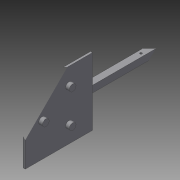
# Autodesk Inventor part: Arm_Base-Rod-Rev2
Saved by Autodesk Inventor 2015 (Build 190159000, 159)
## iProperties
Created: 2016-12-23
Part Number: Arm_Base-Rod-Rev2
Material: Generic
Document SubType Name: Modeling
Designer: Guy
Density: 1 g/cm^3
Appearance: Default
Author: Guy
Autodesk Inventor part; units mm, degrees
ref_plane "YZ Plane" through (0, 0, 0) normal (1, 0, 0) x (0, 1, 0)
ref_plane "XZ Plane" through (0, 0, 0) normal (0, 1, 0) x (-1, 0, 0)
ref_plane "XY Plane" through (0, 0, 0) normal (0, 0, 1) x (1, 0, 0)
sketch "Sketch1" plane through (0, 0, 0) normal (1, 0, 0) x (0, 1, 0)
  line L0 (0, 0) -> (200, 0)
  line L1 (200, 0) -> (200, -200)
  line L2 (200, -200) -> (0, -200)
  line L3 (0, -200) -> (0, 0)
  dimension "d0" = 200
  dimension "d1" = 200
  constraints: 8 end point, 2 parallel, 1 horizontal, 1 perpendicular
  measures "d0" distance of L0.end L1.end
  measures "d1" distance of L0.start L0.end
extrude "Extrusion1" add sketch "Sketch1" along normal blind 6
sketch "Sketch2" plane through (6, 0, 0) normal (1, 0, 0) x (0, 0, -1)
  line L0 (0, 200) -> (0, 0) projected
  line L1 (0, 0) -> (200, 0) projected
  line L2 (200, 0) -> (200, 200) projected
  line L3 (200, 200) -> (0, 200) projected
  circle A0 centre (50, 130) radius 10
  circle A1 centre (150, 130) radius 10
  circle A2 centre (100, 50) radius 10
  dimension "d4" = 20
  dimension "d5" = 20
  dimension "d6" = 20
  dimension "d7" = 100
  dimension "d8" = 50
  dimension "d9" = 80
  dimension "d10" = 100
  dimension "d11" = 50
  dimension "d12" = 80
  constraints: 3 centre point
  measures "d4" diameter of A1
  measures "d5" diameter of A0
  measures "d6" diameter of A2
  measures "d7" distance of A1.centre A0.centre
  measures "d8" distance from line of L2 A1.centre
  measures "d9" vertical distance of A2.centre A0.centre
  measures "d10" distance from line of L2 A2.centre
  measures "d11" distance from line of L1 A2.centre
  measures "d12" vertical distance of A2.centre A1.centre
extrude "Extrusion2" add sketch "Sketch2" along normal blind 11.1 contours A0 | A1 | A2
sketch "Sketch3" plane through (0, 0, 0) normal (-1, 0, 0) x (0, 0, 1)
  line L0 (0, 0) -> (0, 200) projected
  line L1 (0, 200) -> (-200, 200) projected
  line L2 (-200, 200) -> (-200, 0) projected
  line L3 (-200, 0) -> (0, 0) projected
  line L4 (-110, 110) -> (-90, 110)
  line L5 (-90, 110) -> (-90, 90)
  line L6 (-90, 90) -> (-110, 90)
  line L7 (-110, 90) -> (-110, 110)
  dimension "d15" = 20
  dimension "d16" = 20
  dimension "d17" = 90
  dimension "d18" = 90
  constraints: 8 end point, 2 parallel, 1 horizontal, 1 perpendicular
  measures "d15" distance between parallel lines of L5 L7
  measures "d16" distance between parallel lines of L6 L4
  measures "d17" distance between parallel lines of L0 L5
  measures "d18" distance between parallel lines of L3 L6
extrude "Extrusion3" add sketch "Sketch3" along normal blind 20 contours L4 L5 L6 L7
sketch "Sketch4" plane through (0, 110, -90) normal (0, 1, 0) x (1, 0, 0)
  line L0 (0, 20) -> (0, 0) projected
  line L1 (0, 20) -> (-20, 20) projected
  line L2 (-20, 0) -> (-20, 20) projected
  line L3 (0, 0) -> (-20, 0) projected
  line L4 (-20, 0) -> (0, 0)
  line L5 (0, 0) -> (0, 20)
  line L6 (0, 20) -> (-20, 20)
  line L7 (-20, 20) -> (-20, 0)
  point P0 (0, -90)
  constraints: 8 end point, 2 parallel, 1 horizontal, 1 perpendicular
extrude "Extrusion4" add sketch "Sketch4" along normal blind 290
sketch "Sketch5" plane through (-20, 90, -90) normal (0, 0, 1) x (1, 0, 0)
  line L0 (20, 110) -> (20, 0) projected
  line L1 (20, 110) -> (20, 310) projected
  line L2 (0, 310) -> (20, 310) projected
  line L3 (0, 0) -> (0, 310) projected
  line L4 (20, 0) -> (0, 0) projected
  circle A0 centre (10, 270) radius 3.25
  point P0 (20, -90)
  dimension "d23" = 6.5
  dimension "d24" = 40
  dimension "d25" = 10
  constraints: 1 centre point
  measures "d23" diameter of A0
  measures "d24" distance from line of L2 A0.centre
  measures "d25" distance from line of L3 A0.centre
extrude "Extrusion5" cut sketch "Sketch5" against normal up to next contours A0
body "Solid1"
